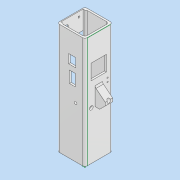
# Autodesk Inventor part: Hull_REV3
Saved by Autodesk Inventor 2020.3 (Build 243373000, 373)
## iProperties
Created: 2020-06-01
Part Number: Hull_REV3
Material: ABS Plastic
Document SubType Name: Modeling
Designer: Derek Wider
Density: 1.06 g/cm^3
Appearance: Smooth - White
Author: Derek Wider
Autodesk Inventor part; units mm, degrees
ref_plane "YZ Plane" through (0, 0, 0) normal (1, 0, 0) x (0, 1, 0)
ref_plane "XZ Plane" through (0, 0, 0) normal (0, 1, 0) x (-1, 0, 0)
sketch "Sketch1" plane through (0, 0, 0) normal (0, 1, 0) x (-1, 0, 0)
  line L0 (3.175, 0) -> (34.925, 0)
  line L1 (38.1, -3.175) -> (38.1, -34.925)
  line L2 (34.925, -38.1) -> (3.175, -38.1)
  line L3 (0, -34.925) -> (0, -3.175)
  line L4 (5.715, -2.54) -> (32.385, -2.54)
  line L5 (35.56, -5.715) -> (35.56, -32.385)
  line L6 (32.385, -35.56) -> (5.715, -35.56)
  line L7 (2.54, -32.385) -> (2.54, -5.715)
  arc A0 (35.56, -5.715) -> (32.385, -2.54) centre (32.385, -5.715) ccw
  arc A1 (38.1, -3.175) -> (34.925, 0) centre (34.925, -3.175) ccw
  arc A2 (32.385, -35.56) -> (35.56, -32.385) centre (32.385, -32.385) ccw
  arc A3 (34.925, -38.1) -> (38.1, -34.925) centre (34.925, -34.925) ccw
  arc A4 (0, -34.925) -> (3.175, -38.1) centre (3.175, -34.925) ccw
  arc A5 (2.54, -32.385) -> (5.715, -35.56) centre (5.715, -32.385) ccw
  arc A6 (5.715, -2.54) -> (2.54, -5.715) centre (5.715, -5.715) ccw
  arc A7 (3.175, 0) -> (0, -3.175) centre (3.175, -3.175) ccw
  point P0 (0, 0)
  point P1 (38.1, -38.1)
  point P2 (38.1, 0)
  point P3 (0, -38.1)
  dimension "d0" = 38.1
  dimension "d1" = 38.1
  dimension "d2" = 2.54
  dimension "d3" = 3.175
  constraints: 16 end point, 16 point on circle, 16 tangent, 8 centre point, 8 point on line, 7 equal radius, 4 parallel, 2 perpendicular, 1 horizontal, 3 other
  measures "d0" distance of point (38.1, -38.1) point (0, -38.1)
  measures "d1" distance of point (38.1, 0) point (38.1, -38.1)
  measures "d2" distance between parallel lines of L3 L7
  measures "d3" radius of A0
extrude "Extrusion1" add sketch "Sketch1" along normal blind 152.4
sketch "Sketch2" plane through (0, 152.4, 0) normal (0, 1, 0) x (1, 0, 0)
  line L0 (-5.715, 2.54) -> (-32.385, 2.54) projected
  line L1 (-32.385, 35.56) -> (-5.715, 35.56) projected
  line L2 (-38.1, 34.925) -> (-38.1, 3.175) projected
  line L3 (-32.385, 2.54) -> (-38.1, 2.54)
  line L4 (-38.1, 2.54) -> (-38.1, 35.56)
  line L5 (-38.1, 35.56) -> (-32.385, 35.56)
  line L6 (-32.385, 35.56) -> (-32.385, 2.54)
  point P0 (0, 0)
  constraints: 8 end point, 2 parallel, 1 horizontal, 1 perpendicular
extrude "Extrusion2" cut sketch "Sketch2" against normal through all
sketch "Sketch3" plane through (0, 152.4, 0) normal (0, 1, 0) x (1, 0, 0)
  line L0 (-38.0359, 35.56) -> (-5.715, 35.56) projected
  arc A0 (-2.54, 32.385) -> (-5.715, 35.56) centre (-5.715, 32.385) ccw projected
  line L1 (-2.54, 32.385) -> (-2.54, 5.715) projected
  arc A1 (-5.715, 2.54) -> (-2.54, 5.715) centre (-5.715, 5.715) ccw projected
  line L2 (-5.715, 2.54) -> (-38.0359, 2.54) projected
  arc A2 (-38.0359, 2.54) -> (-34.925, 0) centre (-34.925, 3.175) ccw projected
  line L3 (-34.925, 0) -> (-3.175, 0) projected
  arc A3 (-3.175, 0) -> (0, 3.175) centre (-3.175, 3.175) ccw projected
  line L4 (0, 3.175) -> (0, 34.925) projected
  arc A4 (0, 34.925) -> (-3.175, 38.1) centre (-3.175, 34.925) ccw projected
  line L5 (-3.175, 38.1) -> (-34.925, 38.1) projected
  arc A5 (-34.925, 38.1) -> (-38.0359, 35.56) centre (-34.925, 34.925) ccw projected
  line L6 (-5.715, 2.54) -> (-38.0359, 2.54) projected
  line L7 (-36.7659, 2.54) -> (-34.2259, 2.54)
  line L8 (-34.2259, 2.54) -> (-34.2259, 3.81)
  line L9 (-34.2259, 3.81) -> (-36.7659, 3.81)
  line L10 (-36.7659, 3.81) -> (-36.7659, 2.54)
  line L11 (-36.7659, 35.56) -> (-34.2259, 35.56)
  line L12 (-34.2259, 35.56) -> (-34.2259, 34.29)
  line L13 (-34.2259, 34.29) -> (-36.7659, 34.29)
  line L14 (-36.7659, 34.29) -> (-36.7659, 35.56)
  point P0 (0, 0)
  dimension "d8" = 2.54
  dimension "d9" = 1.27
  dimension "d10" = 1.27
  constraints: 16 end point, 4 parallel, 2 equal length, 2 horizontal, 2 perpendicular, 2 point on line, 1 vertical alignment
  measures "d8" distance of L9.end L8.end
  measures "d9" distance of L8.end L7.end
  measures "d10" horizontal distance of L9.end L2.end
extrude "Extrusion3" add sketch "Sketch3" against normal up to surface (152.4 mm away) contours L0 L12 L13 L14 | L2 L10 L9 L8
fillet "Fillet1" radius 3.175 2 edges at (-34.2259, 76.2, -35.56) (-34.2259, 76.2, -2.54)
sketch "Sketch5" plane through (0, 152.4, 0) normal (0, 1, 0) x (1, 0, 0)
  line L0 (-36.7659, 2.54) -> (-38.0359, 2.54) projected
  line L1 (-38.0359, 35.56) -> (-36.7659, 35.56) projected
  arc A0 (-38.0359, 2.54) -> (-34.925, 0) centre (-34.925, 3.175) ccw projected
  line L2 (-36.7659, 34.29) -> (-36.7659, 35.56) projected
  line L3 (-38.0359, 2.54) -> (-36.7659, 2.54)
  line L4 (-36.7659, 2.54) -> (-36.7659, 35.56)
  line L5 (-36.7659, 35.56) -> (-38.0359, 35.56)
  line L6 (-38.0359, 35.56) -> (-38.0359, 2.54)
  point P0 (0, 0)
  constraints: 8 end point, 2 parallel, 1 horizontal, 1 perpendicular
extrude "Extrusion4" add sketch "Sketch5" against normal blind 25.4
sketch "Sketch6" plane through (0, 0, -3.175) normal (1, 0, 0) x (0, 0, -1)
  line L0 (0, 152.4) -> (31.75, 152.4) projected
  line L1 (0, 0) -> (0, 152.4) projected
  point P0 (-3.175, 0)
  point P1 (15.875, 76.2)
sketch "Sketch7" plane through (-2.54, 0, -32.385) normal (-1, 0, 0) x (0, 0, 1)
  line L0 (0, 0) -> (26.67, 0) projected
  line L1 (0, 0) -> (0, 152.4) projected
  point P0 (32.385, 0)
  point P1 (13.335, 76.2)
sketch "Sketch8" plane through (-38.0359, 152.4, -35.56) normal (-1, 0, 0) x (0, 0, 1)
  circle A0 centre (24.2706, -10.2436) radius 2.921
  point P0 (35.56, -152.4)
  dimension "d16" = 5.842
  constraints: 1 centre point
  measures "d16" diameter of A0
extrude "Extrusion5" cut sketch "Sketch8" against normal up to surface (1.27 mm away)
sketch "Sketch9" plane through (0, 0, -3.175) normal (1, 0, 0) x (0, 0, -1)
  line L0 (26.375, 119.38) -> (5.375, 119.38)
  line L1 (5.375, 119.38) -> (5.375, 98.3742)
  line L2 (5.375, 98.3742) -> (26.375, 98.3742)
  line L3 (26.375, 98.3742) -> (26.375, 119.38)
  line L4 (0, 152.4) -> (31.75, 152.4) projected
  point P0 (-3.175, 0)
  point P1 (15.875, 119.38)
  point P2 (15.875, 152.4)
  dimension "d19" = 21
  dimension "d20" = 21.0058
  dimension "d21" = 33.02
  constraints: 8 end point, 2 midpoint, 2 parallel, 1 horizontal, 1 perpendicular, 1 vertical alignment
  measures "d19" distance of L2.end L1.end
  measures "d20" distance of L1.end L0.end
  measures "d21" distance between parallel lines of L0 L4
extrude "Extrusion6" cut sketch "Sketch9" against normal up to surface (2.54 mm away)
sketch "Sketch10" plane through (-38.0359, 152.4, -35.56) normal (-1, 0, 0) x (0, 0, 1)
  circle A0 centre (6.8122, -6.6748) radius 1.27
  point P0 (35.56, -152.4)
  dimension "d24" = 2.54
  constraints: 1 centre point
  measures "d24" diameter of A0
extrude "Extrusion7" cut sketch "Sketch10" against normal up to surface (1.27 mm away)
sketch "Sketch11" plane through (-34.925, 0, 0) normal (0, 0, 1) x (1, 0, 0)
  line L0 (12.573, 111.76) -> (22.225, 111.76)
  line L1 (22.225, 111.76) -> (22.225, 123.952)
  line L2 (22.225, 123.952) -> (12.573, 123.952)
  line L3 (12.573, 123.952) -> (12.573, 111.76)
  line L4 (34.925, 0) -> (34.925, 152.4) projected
  dimension "d27" = 9.652
  dimension "d28" = 12.192
  dimension "d52" = 12.7
  dimension "d53" = 111.76
  constraints: 8 end point, 2 parallel, 1 horizontal, 1 perpendicular
  measures "d27" distance of L2.end L1.end
  measures "d28" distance of L1.end L0.end
  measures "d52" distance from line of L4 L0.end
  measures "d53" vertical distance of L4.start L0.end
extrude "Extrusion8" cut sketch "Sketch11" against normal up to surface (2.54 mm away)
sketch "Sketch12" plane through (-34.925, 0, 0) normal (0, 0, 1) x (1, 0, 0)
  circle A0 centre (22.225, 69.85) radius 1.8415
  line L0 (34.925, 0) -> (34.925, 152.4) projected
  dimension "d31" = 3.683
  dimension "d32" = 69.85
  dimension "d33" = 12.7
  constraints: 1 centre point
  measures "d31" diameter of A0
  measures "d32" vertical distance of A0.centre L0.start
  measures "d33" distance from line of L0 A0.centre
extrude "Extrusion9" cut sketch "Sketch12" against normal up to surface (38.1 mm away)
sketch "Sketch13" plane through (-5.715, 0, -2.54) normal (0, 0, -1) x (-1, 0, 0)
  circle A0 centre (6.985, 69.85) radius 1.8415 projected
  line L0 (6.985, 73.8095) -> (10.414, 71.8297)
  line L1 (10.414, 71.8297) -> (10.414, 67.8703)
  line L2 (10.414, 67.8703) -> (6.985, 65.8905)
  line L3 (6.985, 65.8905) -> (3.556, 67.8703)
  line L4 (3.556, 67.8703) -> (3.556, 71.8297)
  line L5 (3.556, 71.8297) -> (6.985, 73.8095)
  line L6 (6.985, 75.1293) -> (11.557, 72.4896)
  line L7 (11.557, 72.4896) -> (11.557, 67.2104)
  line L8 (11.557, 67.2104) -> (6.985, 64.5707)
  line L9 (6.985, 64.5707) -> (2.413, 67.2104)
  line L10 (2.413, 67.2104) -> (2.413, 72.4896)
  line L11 (2.413, 72.4896) -> (6.985, 75.1293)
  point P0 (-5.715, 0)
  dimension "d36" = 6.858
  dimension "d37" = 9.144
  constraints: 24 end point, 2 coincident, 1 parallel, 1 vertical, 26 other
  measures "d36" distance between parallel lines of L4 L1
  measures "d37" distance between parallel lines of L10 L7
extrude "Extrusion10" add sketch "Sketch13" along normal blind 1.905 contours L6 L7 L8 L9 L10 L11
chamfer "Chamfer1" distance 1.905 angle 45 6 edges at (-17.272, 69.85, -2.54) (-14.986, 65.8905, -2.54) (-10.414, 65.8905, -2.54) (-8.128, 69.85, -2.54) (-10.414, 73.8095, -2.54) (-14.986, 73.8095, -2.54)
sketch "Sketch14" plane through (-5.715, 0, -35.56) normal (0, 0, 1) x (1, 0, 0)
  circle A0 centre (-6.985, 69.85) radius 1.8415 projected
  line L0 (-10.414, 67.8703) -> (-10.414, 71.8297)
  line L1 (-10.414, 71.8297) -> (-6.985, 73.8095)
  line L2 (-6.985, 73.8095) -> (-3.556, 71.8297)
  line L3 (-3.556, 71.8297) -> (-3.556, 67.8703)
  line L4 (-3.556, 67.8703) -> (-6.985, 65.8905)
  line L5 (-6.985, 65.8905) -> (-10.414, 67.8703)
  line L6 (-11.557, 67.2104) -> (-11.557, 72.4896)
  line L7 (-11.557, 72.4896) -> (-6.985, 75.1293)
  line L8 (-6.985, 75.1293) -> (-2.413, 72.4896)
  line L9 (-2.413, 72.4896) -> (-2.413, 67.2104)
  line L10 (-2.413, 67.2104) -> (-6.985, 64.5707)
  line L11 (-6.985, 64.5707) -> (-11.557, 67.2104)
  point P0 (5.715, 0)
  dimension "d43" = 6.858
  dimension "d44" = 9.144
  constraints: 24 end point, 2 coincident, 1 parallel, 1 vertical, 26 other
  measures "d43" distance between parallel lines of L3 L0
  measures "d44" distance between parallel lines of L6 L9
extrude "Extrusion11" add sketch "Sketch14" along normal blind 1.905 contours L6 L7 L8 L9 L10 L11
chamfer "Chamfer2" distance 1.905 angle 45 6 edges at (-17.272, 69.85, -35.56) (-14.986, 65.8905, -35.56) (-14.986, 73.8095, -35.56) (-10.414, 65.8905, -35.56) (-8.128, 69.85, -35.56) (-10.414, 73.8095, -35.56)
sketch "Sketch16" plane through (-34.925, 0, 0) normal (0, 0, 1) x (1, 0, 0)
  line L0 (21.717, 104.902) -> (13.716, 104.902)
  line L1 (13.716, 104.902) -> (13.716, 88.9)
  line L2 (13.716, 88.9) -> (21.717, 88.9)
  line L3 (21.717, 88.9) -> (21.717, 104.902)
  line L4 (34.925, 0) -> (34.925, 152.4) projected
  dimension "d50" = 16.002
  dimension "d51" = 8.001
  dimension "d54" = 13.208
  dimension "d55" = 88.9
  constraints: 8 end point, 2 parallel, 1 horizontal, 1 perpendicular
  measures "d50" distance of L0.end L1.end
  measures "d51" distance of L1.end L2.end
  measures "d54" distance from line of L4 L2.end
  measures "d55" vertical distance of L4.start L2.end
extrude "Extrusion12" cut sketch "Sketch16" against normal up to surface (2.54 mm away)
sketch "Sketch17" plane through (0, 0, -3.175) normal (1, 0, 0) x (0, 0, -1)
  line L0 (10.795, 65.0875) -> (20.955, 65.0875)
  line L1 (20.955, 65.0875) -> (20.955, 87.3125)
  line L2 (20.955, 87.3125) -> (10.795, 87.3125)
  line L3 (10.795, 87.3125) -> (10.795, 65.0875)
  line L4 (0, 0) -> (31.75, 0) projected
  line L5 (34.925, 0) -> (34.925, 152.4) projected
  point P0 (-3.175, 0)
  point P1 (15.875, 65.0875)
  point P2 (15.875, 0)
  point P3 (10.795, 76.2)
  point P4 (34.925, 76.2)
  dimension "d58" = 10.16
  dimension "d59" = 22.225
  constraints: 8 end point, 4 midpoint, 2 parallel, 1 horizontal, 1 horizontal alignment, 1 perpendicular, 1 vertical alignment
  measures "d58" distance of L2.end L1.end
  measures "d59" distance of L1.end L0.end
extrude "Extrusion13" add sketch "Sketch17" along normal blind 13.97
chamfer "Chamfer3" distance 10.16 distance2 12.7 1 edges at (13.97, 87.3125, -19.05) measured on face at (13.97, 72.4958, -20.7433)
sketch "Sketch18" plane through (13.97, 0, -3.175) normal (1, 0, 0) x (0, 0, -1)
  line L0 (0, 0) -> (0, 152.4) projected
  line L1 (10.795, 77.1525) -> (20.955, 77.1525) projected
  line L2 (10.795, 77.1525) -> (10.795, 65.0875) projected
  line L3 (10.795, 65.0875) -> (20.955, 65.0875) projected
  line L4 (20.955, 65.0875) -> (20.955, 77.1525) projected
  circle A0 centre (15.875, 76.2) radius 2.54
  point P0 (-3.175, 0)
  dimension "d65" = 5.08
  constraints: 1 centre point
  measures "d65" diameter of A0
ref_plane "Work Plane1" through (-5.715, 0, -19.05) normal (0, 0, -1) x (-1, 0, 0)
sketch "Sketch19" plane through (-5.715, 0, -19.05) normal (0, 0, -1) x (-1, 0, 0)
  line L0 (-5.715, 0) -> (-5.715, 152.4) projected
  line L1 (-19.685, 65.0875) -> (-19.685, 77.1525) projected
  line L2 (-5.715, 65.0875) -> (-19.685, 65.0875) projected
  arc A0 (-8.5725, 65.0875) -> (-19.685, 76.2) centre (-19.685, 65.0875) ccw
  point P0 (-5.715, 76.2)
  constraints: 2 line through centre, 2 point on circle, 2 point on line, 1 centre point, 1 horizontal alignment, 1 midpoint
sweep "Sweep1" cut profiles "Sketch18" path "Sketch19" path curves A0 contours A0 L1 | L1 A0
chamfer "Chamfer4" distance 7.62 angle 45 1 edges at (13.97, 65.0875, -19.05)
sketch "Sketch20" plane through (0, 0, -3.175) normal (1, 0, 0) x (0, 0, -1)
  circle A0 centre (5.715, 66.04) radius 2.54
  line L0 (0, 0) -> (31.75, 0) projected
  line L1 (0, 0) -> (0, 152.4) projected
  point P0 (-3.175, 0)
  point P1 (15.875, 0)
  dimension "d71" = 5.08
  dimension "d75" = 5.715
  dimension "d76" = 66.04
  constraints: 1 centre point, 1 midpoint
  measures "d71" diameter of A0
  measures "d75" distance from line of L1 A0.centre
  measures "d76" distance from line of L0 A0.centre
extrude "Extrusion14" cut sketch "Sketch20" against normal blind 25.4
sketch "Sketch21" plane through (0, 0, -3.175) normal (1, 0, 0) x (0, 0, -1)
  line L0 (20.955, 65.0875) -> (10.795, 65.0875) projected
  line L1 (19.05, 65.0875) -> (31.75, 65.0875)
  line L2 (31.75, 65.0875) -> (31.75, 58.9915)
  line L3 (31.75, 58.9915) -> (19.05, 58.9915)
  line L4 (19.05, 58.9915) -> (19.05, 65.0875)
  line L5 (31.75, 0) -> (31.75, 152.4) projected
  point P0 (-3.175, 0)
  dimension "d77" = 12.7
  dimension "d78" = 6.096
  constraints: 8 end point, 2 parallel, 2 point on line, 1 horizontal, 1 perpendicular
  measures "d77" distance of L2.end L3.end
  measures "d78" distance of L1.end L2.end
extrude "Extrusion15" cut sketch "Sketch21" against normal blind 7.62
sketch "Sketch22" plane through (-2.54, 0, -32.385) normal (-1, 0, 0) x (0, 0, 1)
  circle A0 centre (1.27, 90.811) radius 0.889
  circle A1 centre (1.27, 85.731) radius 0.889
  line L0 (0, 65.0875) -> (0, 152.4) projected
  point P0 (32.385, 0)
  dimension "d81" = 1.778
  dimension "d82" = 1.778
  dimension "d83" = 5.08
  dimension "d84" = 1.27
  constraints: 2 centre point, 1 vertical alignment
  measures "d81" diameter of A0
  measures "d82" diameter of A1
  measures "d83" distance of A0.centre A1.centre
  measures "d84" distance from line of A1.centre L0
extrude "Extrusion16" cut sketch "Sketch22" against normal blind 25.4
fillet "Fillet2" radius 3.175 1 edges at (0, 87.3125, -19.05)
sketch "Sketch23" plane through (-34.925, 0, 0) normal (0, 0, 1) x (1, 0, 0)
  line L0 (13.716, 104.902) -> (21.717, 104.902) projected
  line L1 (21.717, 104.902) -> (21.717, 88.9) projected
  line L2 (21.717, 88.9) -> (13.716, 88.9) projected
  line L3 (13.716, 88.9) -> (13.716, 104.902) projected
  circle A0 centre (22.225, 69.85) radius 1.8415 projected
  line L4 (22.225, 111.76) -> (12.573, 111.76) projected
  line L5 (12.573, 111.76) -> (12.573, 123.952) projected
  line L6 (12.573, 123.952) -> (22.225, 123.952) projected
  line L7 (22.225, 123.952) -> (22.225, 111.76) projected
  line L8 (0, 0) -> (31.75, 0) projected
  line L9 (31.75, 0) -> (31.75, 152.4) projected
  line L10 (0, 152.4) -> (31.75, 152.4) projected
  line L11 (0, 0) -> (0, 152.4) projected
  line L12 (12.573, 111.76) -> (22.225, 111.76) projected
  line L13 (12.573, 123.952) -> (22.225, 123.952) projected
  line L14 (18.0589, 111.76) -> (16.3269, 111.76)
  line L15 (16.3269, 111.76) -> (16.3269, 123.952)
  line L16 (16.3269, 123.952) -> (18.0589, 123.952)
  line L17 (18.0589, 123.952) -> (18.0589, 111.76)
  line L18 (21.717, 88.9) -> (13.716, 88.9) projected
  line L19 (18.9033, 88.9) -> (16.3269, 88.9)
  line L20 (16.3269, 88.9) -> (16.3269, 104.902)
  line L21 (16.3269, 104.902) -> (18.9033, 104.902)
  line L22 (18.9033, 104.902) -> (18.9033, 88.9)
  point P0 (34.925, 0)
  constraints: 16 end point, 4 parallel, 4 point on line, 2 horizontal, 2 perpendicular
extrude "Extrusion17" [suppressed]
sketch "Sketch24" plane through (0, 0, -3.175) normal (1, 0, 0) x (0, 0, -1)
  line L0 (20.955, 89.8525) -> (20.955, 65.0875) projected
  line L1 (20.955, 65.0875) -> (31.75, 65.0875) projected
  line L2 (31.75, 65.0875) -> (31.75, 152.4) projected
  line L3 (0, 152.4) -> (31.75, 152.4) projected
  line L4 (0, 0) -> (0, 152.4) projected
  line L5 (0, 0) -> (31.75, 0) projected
  line L6 (31.75, 0) -> (31.75, 58.9915) projected
  line L7 (31.75, 58.9915) -> (19.05, 58.9915) projected
  line L8 (19.05, 58.9915) -> (19.05, 65.0875) projected
  line L9 (19.05, 65.0875) -> (10.795, 65.0875) projected
  line L10 (10.795, 65.0875) -> (10.795, 89.8525) projected
  line L11 (20.955, 89.8525) -> (10.795, 89.8525) projected
  circle A0 centre (27.94, 85.731) radius 0.889 projected
  circle A1 centre (27.94, 90.811) radius 0.889 projected
  line L12 (5.375, 119.38) -> (26.375, 119.38) projected
  line L13 (26.375, 119.38) -> (26.375, 98.3742) projected
  line L14 (26.375, 98.3742) -> (5.375, 98.3742) projected
  line L15 (5.375, 98.3742) -> (5.375, 119.38) projected
  circle A2 centre (5.715, 66.04) radius 2.54 projected
  line L16 (26.375, 98.3742) -> (5.375, 98.3742) projected
  line L17 (5.375, 119.38) -> (26.375, 119.38) projected
  line L18 (23.9436, 98.3742) -> (22.8356, 98.3742)
  line L19 (22.8356, 98.3742) -> (22.8356, 119.38)
  line L20 (22.8356, 119.38) -> (23.9436, 119.38)
  line L21 (23.9436, 119.38) -> (23.9436, 98.3742)
  line L22 (20.0658, 98.3742) -> (18.0082, 98.3742)
  line L23 (18.0082, 98.3742) -> (18.0082, 119.38)
  line L24 (18.0082, 119.38) -> (20.0658, 119.38)
  line L25 (20.0658, 119.38) -> (20.0658, 98.3742)
  line L26 (14.9225, 98.3742) -> (12.9434, 98.3742)
  line L27 (12.9434, 98.3742) -> (12.9434, 119.38)
  line L28 (12.9434, 119.38) -> (14.9225, 119.38)
  line L29 (14.9225, 119.38) -> (14.9225, 98.3742)
  line L30 (10.0153, 98.3742) -> (8.255, 98.3742)
  line L31 (8.255, 98.3742) -> (8.255, 119.38)
  line L32 (8.255, 119.38) -> (10.0153, 119.38)
  line L33 (10.0153, 119.38) -> (10.0153, 98.3742)
  line L34 (31.75, 58.9915) -> (19.05, 58.9915) projected
  line L35 (20.955, 65.0875) -> (31.75, 65.0875) projected
  line L36 (21.985, 58.9915) -> (23.3896, 58.9915)
  line L37 (23.3896, 58.9915) -> (23.3896, 65.0875)
  line L38 (23.3896, 65.0875) -> (21.985, 65.0875)
  line L39 (21.985, 65.0875) -> (21.985, 58.9915)
  line L40 (27.94, 58.9915) -> (29.409, 58.9915)
  line L41 (29.409, 58.9915) -> (29.409, 65.0875)
  line L42 (29.409, 65.0875) -> (27.94, 65.0875)
  line L43 (27.94, 65.0875) -> (27.94, 58.9915)
  point P0 (-3.175, 0)
  constraints: 48 end point, 12 parallel, 12 point on line, 6 horizontal, 6 perpendicular
extrude "Extrusion18" [suppressed]
body "Solid1"
